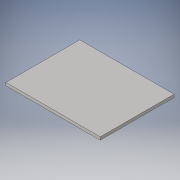
# Autodesk Inventor part: Top
Saved by Autodesk Inventor 2016 (Build 200138000, 138)
## iProperties
Created: 2017-10-30
Part Number: Top
Material: Generic
Document SubType Name: Modeling
Designer: mathaetaes
Density: 1 g/cm^3
Appearance: Default
Author: mathaetaes
Autodesk Inventor part; units mm, degrees
ref_plane "YZ Plane" through (0, 0, 0) normal (1, 0, 0) x (0, 1, 0)
ref_plane "XZ Plane" through (0, 0, 0) normal (0, 1, 0) x (-1, 0, 0)
ref_plane "XY Plane" through (0, 0, 0) normal (0, 0, 1) x (1, 0, 0)
sketch "Sketch1" plane through (0, 0, 0) normal (0, 1, 0) x (-1, 0, 0)
  line L0 (386.9283, -286.643) -> (-432.2217, -286.643)
  line L1 (-432.2217, -286.643) -> (-432.2217, 354.707)
  line L2 (-432.2217, 354.707) -> (386.9283, 354.707)
  line L3 (386.9283, 354.707) -> (386.9283, -286.643)
  point P0 (0, 0)
  dimension "d0" = 641.35
  dimension "d1" = 819.15
  constraints: 8 end point, 2 parallel, 1 horizontal, 1 perpendicular
  measures "d0" distance of L0.end L1.end
  measures "d1" distance of L1.end L2.end
extrude "Board" add sketch "Sketch1" along normal blind 25.4
sketch "Sketch2" plane through (0, 0, 0) normal (0, -1, 0) x (1, 0, 0)
  line L0 (422.6967, -286.643) -> (413.1717, -286.643)
  line L1 (413.1717, -286.643) -> (413.1717, 183.257)
  line L2 (413.1717, 183.257) -> (422.6967, 183.257)
  line L3 (422.6967, 183.257) -> (422.6967, -286.643)
  line L4 (-367.8783, -286.643) -> (-377.4033, -286.643)
  line L5 (-377.4033, -286.643) -> (-377.4033, 183.257)
  line L6 (-377.4033, 183.257) -> (-367.8783, 183.257)
  line L7 (-367.8783, 183.257) -> (-367.8783, -286.643)
  line L8 (-386.9283, -286.643) -> (432.2217, -286.643) projected
  line L9 (432.2217, -286.643) -> (432.2217, 354.707) projected
  line L10 (-386.9283, -286.643) -> (-386.9283, 354.707) projected
  line L11 (13.1217, -286.643) -> (32.1717, -286.643)
  line L12 (32.1717, -286.643) -> (32.1717, 183.257)
  line L13 (32.1717, 183.257) -> (13.1217, 183.257)
  line L14 (13.1217, 183.257) -> (13.1217, -286.643)
  point P0 (0, 0)
  dimension "d4" = 469.9
  dimension "d5" = 9.525
  dimension "d6" = 9.525
  dimension "d7" = 9.525
  dimension "d10" = 19.05
  dimension "d11" = 819.15
  dimension "d12" = 400.05
  dimension "d14" = 400.05
  constraints: 24 end point, 6 parallel, 4 collinear, 3 horizontal, 3 perpendicular, 2 equal length
  measures "d4" distance of L0.end L1.end
  measures "d5" distance of L1.end L2.end
  measures "d6" distance between parallel lines of L3 L9
  measures "d7" distance between parallel lines of L10 L5
  measures "d10" distance of L13.end L12.end
  measures "d11" distance between parallel lines of L9 L10
  measures "d12" distance between parallel lines of L14 L10
  measures "d14" distance between parallel lines of L9 L12
extrude "Vertical Wall Stop Dado Notches" cut sketch "Sketch2" against normal blind 12.7
equation "\"d7\" = d6"
equation "\"d12\" = 0.5 * d11 - 0.5 * d10"
body "Solid1"
